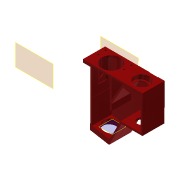
# Autodesk Inventor part: cellSTORM_v5_opticalstage
Saved by Autodesk Inventor 2022 (Build 260153000, 153)
## iProperties
Created: 2020-04-25
Part Number: cellSTORM_v5_opticalstage
Material: Generic
Document SubType Name: Modeling
Designer: diederichbenedict
Density: 1 g/cm^3
Appearance: Red
Author: diederichbenedict
Autodesk Inventor part; units mm, degrees
ref_plane "Work Plane1" through (0, 0, 0) normal (0, 0, 1) x (1, 0, 0)
ref_plane "Work Plane2" through (79.8747, 18.9526, -58.9639) normal (0, 0.0044332, 0.9999902) x (1, 0, 0)
sketch "Sketch2" plane through (79.8747, 18.9526, -58.9639) normal (0, 0.0044332, 0.9999902) x (1, 0, 0)
  line L0 (-7.3391, -43.0706) -> (-11.3391, -43.0706)
  line L1 (-7.3391, -43.0706) -> (-3.3391, -43.0706) construction
  line L2 (-11.3391, -43.0706) -> (-11.3391, -85.3324)
  line L3 (-11.3391, -85.3324) -> (19.5839, -90.7849)
  line L4 (39.6609, -51.3324) -> (73.6609, -51.3324)
  line L5 (-28.496, 8.6676) -> (-11.3391, 8.6676)
  line L6 (-11.3391, 8.6676) -> (-11.3391, -43.0706)
  line L7 (19.5839, -90.7849) -> (39.6609, -51.3324)
  line L8 (-28.496, 8.6676) -> (73.6609, 8.6676)
  line L9 (73.6609, 8.6676) -> (73.6609, -51.3324)
  line L10 (-7.2559, -79.452) -> (-8.211, -84.8684)
  line L11 (17.7582, -83.8627) -> (16.8031, -89.2791)
  line L12 (38.3797, -66.8653) -> (38.3797, -46.8653) projected
  line L13 (-11.3391, 8.6676) -> (-23.3391, 8.6676)
  line L14 (-23.3391, 8.6676) -> (-23.3391, 3.6676)
  line L15 (-23.3391, 3.6676) -> (-11.3391, 3.6676)
  line L16 (-11.3391, 3.6676) -> (-11.3391, 8.6676)
  ellipse E0 centre (54.5234, 5.3365) end of major axis (42.0164, 7.5419) minor radius 0.0004 projected
  ellipse E1 centre (3.9219, -87.5114) end of major axis (-8.339, -85.3495) minor radius 0.0004 projected
  point P0 (-79.8747, -19.2138)
  point P1 (-11.3391, 3.6676)
  point P2 (-23.3391, 8.6676)
  dimension "d0" = 4
  dimension "d1" = 180
  dimension "d156" = 3
  dimension "d157" = 3
  dimension "d158" = 1
  dimension "d159" = 94
  dimension "d160" = 85
  dimension "d161" = 60
  dimension "d163" = 34
  dimension "d180" = 12
  dimension "d181" = 5
  constraints: 32 end point, 5 horizontal, 3 parallel, 2 collinear, 2 perpendicular, 1 vertical, 9 other
  measures "d0" distance of L0.start L0.end
  measures "d1" angle of L0 L1
  measures "d156" distance from line of L2.end L10
  measures "d157" distance from line of L3.end L11
  measures "d158" distance from line of L3 L11.end
  measures "d159" distance from line of L8 L2.end
  measures "d160" distance between parallel lines of L9 L6
  measures "d161" distance between parallel lines of L8 L4
  measures "d163" distance from line of L9 L4.start
  measures "d180" distance of L15.end L14.end
  measures "d181" distance of L14.end L13.end
extrude "Extrusion1" add sketch "Sketch2" along normal blind 4 contours L6 L8 L9 L4 L7 L3 L2 | L15 L14 L5 L6 | E0 | E1
sketch "Sketch3" plane through (79.8747, 18.9703, -54.964) normal (0, 0.0044332, 0.9999902) x (1, 0, 0)
  line L0 (73.6609, 8.6676) -> (-23.3391, 8.6676) projected
  line L1 (-11.3391, 3.6676) -> (-11.3391, -85.3324) projected
  line L2 (-11.3391, -85.3324) -> (19.5839, -90.7849) projected
  line L3 (19.5839, -90.7849) -> (39.6609, -51.3324) projected
  line L4 (39.6609, -51.3324) -> (73.6609, -51.3324) projected
  line L5 (73.6609, -51.3324) -> (73.6609, 8.6676) projected
  line L6 (70.6609, 5.6676) -> (-8.3391, 5.6676)
  line L7 (-8.3391, 5.6676) -> (-8.3391, -82.8151)
  line L8 (-8.3391, -82.8151) -> (17.9175, -87.4448)
  line L9 (17.9175, -87.4448) -> (37.8215, -48.3324)
  line L10 (37.8215, -48.3324) -> (70.6609, -48.3324)
  line L11 (70.6609, -48.3324) -> (70.6609, 5.6676)
  line L12 (20.3299, 5.6676) -> (20.3299, -36.4597)
  line L13 (20.3299, -36.4597) -> (44.6523, 5.6676)
  line L14 (41.1882, 5.6676) -> (23.3299, -25.2636)
  line L15 (23.3299, -25.2636) -> (23.3299, 5.6676)
  line L16 (50.5927, -0.5756) -> (7.6402, -74.9707)
  line L17 (-23.3391, 8.6676) -> (-23.3391, 3.6676) projected
  line L18 (-23.3391, 3.6676) -> (-11.3391, 3.6676) projected
  line L19 (23.3299, -31.2636) -> (23.3299, -41.2636)
  line L20 (23.3299, -41.2636) -> (20.3299, -41.2636)
  line L21 (20.3299, -41.2636) -> (20.3299, -36.4597)
  point P0 (-79.8747, -19.2138)
  point P1 (-36.2088, 5.0266)
  dimension "d165" = 3
  dimension "d166" = 3
  dimension "d167" = 3
  dimension "d211" = 10
  constraints: 28 end point, 5 point on line, 3 perpendicular, 2 parallel, 2 vertical, 8 other
  measures "d165" distance between parallel lines of L5 L11
  measures "d166" distance between parallel lines of L12 L15
  measures "d167" distance between parallel lines of L13 L14
  measures "d211" distance of L19.start L19.end
extrude "Extrusion2" add sketch "Sketch3" along normal blind 32 contours L5 L4 L3 L2 L1 L18 L17 L0 | L13 L12 L6 L15 L14 | L19 L20 L21 L13
ref_plane "Work Plane3" through (51.6835, -64.2382, -58.0722) normal (0.309017, 0.9510565, 0) x (-0.6726294, 0.2185505, 0.7069691)
ref_plane "Work Plane4" through (49.8294, -69.9446, -58.0722) normal (-0.309017, -0.9510565, 0) x (0.6723676, -0.2184655, 0.7072444)
sketch "Sketch7" plane through (51.6691, -60.1991, -22.6127) normal (0.1736475, 0.9847982, -0.0043659) x (0.9848079, -0.1736458, 0.0007698)
  circle A0 centre (33.264, 17.4442) radius 12
  ellipse E0 centre (33.0632, 17.4064) end of major axis (45.5132, 17.4064) minor radius 12.45 projected
  point P0 (-61.32, -22.8793)
  dimension "d33" = 24
  constraints: 1 centre point
  measures "d33" diameter of A0
extrude "Extrusion5" cut sketch "Sketch7" against normal blind 5 contours A0
ref_plane "Work Plane5" through (122.0405, 25.1021, -58.0722) normal (-0.309017, -0.9510565, 0) x (0.6723676, -0.2184655, 0.7072444)
sketch "Sketch11" plane through (47.2299, 24.6379, -54.9891) normal (0, 0.9999902, -0.0044332) x (1, 0, 0)
  circle A0 centre (37.6585, -14.4614) radius 15.35
  circle A1 centre (-11.9932, -35.7166) radius 13.9 projected
  point P0 (-47.2299, -54.8793)
  dimension "d43" = 30.7
  constraints: 1 centre point
  measures "d43" diameter of A0
extrude "Extrusion9" cut sketch "Sketch11" along normal mid plane 60 contours A0
ref_plane "Arbeitsebene11" through (104.1095, -44.1462, -23.1152) normal (0, -1, 0) x (1, 0, 0)
sketch "Sketch21" plane through (104.1095, -44.1462, -23.1152) normal (0, -1, 0) x (1, 0, 0)
  ellipse E0 centre (30.7788, -17.1459) end of major axis (28.2788, -17.1459) minor radius 2.5 projected
  circle A0 centre (30.7788, -17.1459) radius 7.5
  point P0 (-104.1095, 23.1152)
  dimension "d214" = 15
  constraints: 1 centre point, 1 coincident, 1 other
  measures "d214" diameter of A0
extrude "Extrusion17" cut sketch "Sketch21" against normal blind 15 contours E0 | A0
sketch "Sketch22" plane through (68.5356, -66.3789, -58.5856) normal (-1, 0, 0) x (0, 0.0044332, 0.9999902)
  line L0 (0, 89) -> (0, 0) projected
  line L1 (0, 0) -> (36, 0) projected
  line L2 (4, 109.1334) -> (4, 78) projected
  line L3 (4, 59.5268) -> (36, 59.5268) projected
  line L4 (4, 78) -> (36, 59.5268)
  line L5 (36, 59.5268) -> (4, 59.5268)
  line L6 (4, 78) -> (4, 0) projected
  line L7 (4, 59.5268) -> (4, 78)
  line L8 (36, 89) -> (36, 0) projected
  line L9 (36, 89) -> (0, 89) projected
  point P0 (58.8793, 66.1185)
  constraints: 6 end point, 1 perpendicular
extrude "Extrusion18" add sketch "Sketch22" against normal blind 2 contours L4 L3 L6
sketch "Skizze26" plane through (79.8747, 18.9526, -58.9639) normal (0, -0.0044332, -0.9999902) x (-1, 0, 0)
  circle A0 centre (-56.1499, 7.231) radius 1.75 projected
  circle A1 centre (-56.1499, -2.769) radius 1.75 projected
  circle A2 centre (-56.1499, -12.769) radius 1.75 projected
  circle A3 centre (-56.1499, -22.769) radius 1.75 projected
  point P0 (79.8747, -19.2138)
hole "Bohrung4" at (136.0246, 26.1835, -58.996) direction (0, 0.0044332, 0.9999902) diameter 2.8 depth 12 tip angle 118
pattern_linear "Rechteckige Anordnung1" count 12 spacing 12.5 along (0, -0.9999902, 0.0044332) of "Bohrung4"
sketch "Skizze28" plane through (79.8747, 18.9526, -58.9639) normal (0, -0.0044332, -0.9999902) x (-1, 0, 0)
  line L0 (-50.0499, -35.324) -> (-50.0499, -2.924) projected
  line L1 (-62.0499, -35.324) -> (-62.0499, -2.924) projected
  line L2 (-49.0499, 19.5051) -> (-63.0499, 19.5051)
  line L3 (-63.0499, 19.5051) -> (-63.0499, -40.5846)
  line L4 (-63.0499, -40.5846) -> (-49.0499, -40.5846)
  line L5 (-49.0499, -40.5846) -> (-49.0499, 19.5051)
  point P0 (79.8747, -19.2138)
  dimension "d134" = 1
  dimension "d135" = 1
  constraints: 8 end point, 2 parallel, 1 horizontal, 1 perpendicular
  measures "d134" distance between parallel lines of L0 L5
  measures "d135" distance between parallel lines of L3 L1
extrude "Extrusion21" cut sketch "Skizze28" against normal blind 0.5
sketch "Skizze30" plane through (71.5356, -63.8439, -54.5968) normal (0.1736475, 0.9847982, -0.0043659) x (0.9848079, -0.1736458, 0.0007698)
  circle A0 centre (13.091, -14.5558) radius 12 projected
  line L0 (-2.5173, -32) -> (28.8827, -32) projected
  line L1 (27.091, 2.8884) -> (-0.909, 2.8884)
  line L2 (-0.909, 2.8884) -> (-0.909, -32)
  line L3 (-0.909, -32) -> (27.091, -32)
  line L4 (27.091, -32) -> (27.091, 2.8884)
  line L5 (27.091, 2.8884) -> (-0.909, -32) construction
  line L6 (-0.909, 2.8884) -> (27.091, -32) construction
  circle A1 centre (13.091, -14.5558) radius 12.75
  point P0 (-81.493, -54.8793)
  point P1 (27.091, -32)
  dimension "d168" = 28
  dimension "d171" = 25.5
  constraints: 12 end point, 2 midpoint, 2 parallel, 1 centre point, 1 coincident, 1 horizontal, 1 perpendicular, 1 point on line
  measures "d168" distance of L3.end L2.end
  measures "d171" diameter of A1
extrude "Extrusion23" add sketch "Skizze30" along normal blind 5 contours L2 L1 L4 L0
sketch "Skizze31" plane through (79.8747, 18.9703, -54.964) normal (0, 0.0044332, 0.9999902) x (1, 0, 0)
  line L0 (19.2086, -82.5953) -> (18.5846, -86.1339) projected
  line L1 (18.5846, -86.1339) -> (37.8215, -48.3324) projected
  line L2 (37.8215, -48.3324) -> (70.6609, -48.3324) projected
  line L3 (70.6609, -48.3324) -> (70.6609, 5.6676) projected
  line L4 (70.6609, 5.6676) -> (44.6523, 5.6676) projected
  line L5 (44.6523, 5.6676) -> (23.3299, -31.2636) projected
  line L6 (20.3299, -41.2636) -> (20.3299, 5.6676) projected
  line L7 (20.3299, 5.6676) -> (10.1606, 5.6676) projected
  line L8 (10.1606, 5.6676) -> (10.1606, -24.3324) projected
  line L9 (10.1606, -24.3324) -> (-0.1332, -24.3324) projected
  line L10 (-0.1332, -24.3324) -> (-0.1332, 5.6676) projected
  line L11 (-0.1332, 5.6676) -> (-8.3391, 5.6676) projected
  line L12 (-8.3391, 5.6676) -> (-8.3391, -77.7379) projected
  line L13 (-8.3391, -77.7379) -> (19.2086, -82.5953) projected
  circle A0 centre (56.1499, -30.269) radius 1.4 projected
  circle A1 centre (56.1499, -17.769) radius 1.4 projected
  circle A2 centre (56.1499, -5.269) radius 1.4 projected
  line L14 (-3.3391, -73.5424) -> (-3.3391, -29.3324)
  line L15 (-3.3391, -29.3324) -> (15.1606, -29.3324)
  line L16 (15.1606, -29.3324) -> (15.1606, 0.6676)
  line L17 (15.1606, 0.6676) -> (15.3299, 0.6676)
  line L18 (15.3299, 0.6676) -> (15.3299, -55.1198)
  line L19 (15.3299, -55.1198) -> (47.539, 0.6676)
  line L20 (47.539, 0.6676) -> (65.6609, 0.6676)
  line L21 (65.6609, 0.6676) -> (65.6609, -43.3324)
  line L22 (65.6609, -43.3324) -> (34.7558, -43.3324)
  line L23 (34.7558, -43.3324) -> (17.5112, -77.2189)
  line L24 (17.5112, -77.2189) -> (-3.3391, -73.5424)
  circle A3 centre (56.1499, -42.769) radius 1.4 projected
  line L25 (23.3299, -31.2636) -> (23.3299, -41.2636) projected
  line L26 (23.3299, -41.2636) -> (20.3299, -41.2636) projected
  point P0 (-79.8747, -19.2138)
  dimension "d172" = 5
  constraints: 22 end point, 10 other
  measures "d172" distance between parallel lines of L12 L14
hole "Bohrung5" at (76.5356, -10.3617, -54.8339) at (95.0352, -10.3617, -54.8339) direction (0, -0.0044332, -0.9999902) diameter 3 end through all
sketch "Skizze32" plane through (56.5356, 27.7798, -23.0027) normal (0, 0.9999902, -0.0044332) x (1, 0, 0)
  line L0 (86.3889, 36) -> (86.3889, 35.5) projected
  line L1 (86.3889, 35.5) -> (72.3889, 35.5) projected
  line L2 (72.3889, 35.5) -> (72.3889, 36) projected
  line L3 (72.3889, 36) -> (0, 36) projected
  line L4 (0, 36) -> (0, 0) projected
  line L5 (97, 0) -> (0, 0) projected
  line L6 (97, 36) -> (97, 0) projected
  line L7 (97, 36) -> (86.3889, 36) projected
  circle A0 centre (28.3527, 17.5386) radius 15.35 projected
  circle A1 centre (5.9968, 30.9932) radius 1.4
  circle A2 centre (5.9968, 18.9932) radius 1.4
  circle A3 centre (47.9968, 18.9932) radius 1.4
  circle A4 centre (47.9968, 30.9932) radius 1.4
  point P0 (-56.5356, -22.8793)
  dimension "d182" = 2.8
  dimension "d183" = 2.8
  dimension "d185" = 2.8
  dimension "d186" = 2.8
  dimension "d187" = 12
  dimension "d188" = 12
  dimension "d189" = 0
  dimension "d190" = 42
  dimension "d191" = 0
  dimension "d192" = 0
  constraints: 4 centre point
  measures "d182" diameter of A1
  measures "d183" diameter of A2
  measures "d185" diameter of A3
  measures "d186" diameter of A4
  measures "d187" distance of A4.centre A3.centre
  measures "d188" distance of A2.centre A1.centre
  measures "d189" vertical distance of A4.centre A1.centre
  measures "d190" distance of A4.centre A1.centre
  measures "d191" horizontal distance of A3.centre A4.centre
  measures "d192" horizontal distance of A2.centre A1.centre
extrude "Extrusion24" cut sketch "Skizze32" against normal blind 20 contours A1 | A2 | A3 | A4
sketch "Skizze34" plane through (79.8747, 19.1122, -22.9643) normal (0, 0.0044332, 0.9999902) x (1, 0, 0)
  line L0 (-23.3391, 8.6676) -> (-23.3391, 3.6676) projected
  line L1 (-23.3391, 3.6676) -> (-11.3391, 3.6676) projected
  line L2 (-11.3391, 3.6676) -> (-11.3391, -85.3324) projected
  line L3 (-11.3391, -85.3324) -> (19.5839, -90.7849) projected
  line L4 (19.5839, -90.7849) -> (39.6609, -51.3324) projected
  line L5 (39.6609, -51.3324) -> (73.6609, -51.3324) projected
  line L6 (73.6609, -51.3324) -> (73.6609, 8.6676) projected
  line L7 (73.6609, 8.6676) -> (-23.3391, 8.6676) projected
  line L8 (23.3299, -25.2636) -> (23.3299, 5.6676) projected
  line L9 (23.3299, 5.6676) -> (41.1882, 5.6676) projected
  line L10 (41.1882, 5.6676) -> (23.3299, -25.2636) projected
  line L11 (18.5846, -86.1339) -> (19.2086, -82.5953) projected
  line L12 (-8.3391, -77.7379) -> (19.2086, -82.5953) projected
  line L13 (-8.3391, -77.7379) -> (-8.3391, 5.6676) projected
  line L14 (-8.3391, 5.6676) -> (20.3299, 5.6676) projected
  line L15 (20.3299, 5.6676) -> (20.3299, -41.2636) projected
  line L16 (23.3299, -31.2636) -> (44.6523, 5.6676) projected
  line L17 (44.6523, 5.6676) -> (70.6609, 5.6676) projected
  line L18 (70.6609, 5.6676) -> (70.6609, -48.3324) projected
  line L19 (70.6609, -48.3324) -> (37.8215, -48.3324) projected
  line L20 (37.8215, -48.3324) -> (18.5846, -86.1339) projected
  line L21 (70.6609, 5.6676) -> (70.6609, -48.3324) projected
  line L22 (20.3299, -41.2636) -> (23.3299, -41.2636) projected
  line L23 (23.3299, -41.2636) -> (23.3299, -31.2636) projected
  ellipse E0 centre (53.5684, -0.0799) end of major axis (66.0754, -2.2852) minor radius 0.0004 projected
  line L24 (70.6609, -3.7406) -> (41.8024, 0.7315)
  point P0 (-79.8747, -19.2138)
  dimension "d213" = 1
  constraints: 2 end point, 2 point on line
  measures "d213" distance from line of E0.centre L24
extrude "Extrusion25" add sketch "Skizze34" against normal up to surface (32 mm away) contours L24 L16 L17 L18
sketch "Skizze35" plane through (122.1669, 19.7678, -22.9672) normal (-0.1531354, -0.9881955, 0.0043809) x (0.9882052, -0.1531339, 0.0006789)
  circle A0 centre (11.5094, -17.485) radius 12.7
  circle A1 centre (11.5094, -17.485) radius 10
  ellipse E0 centre (11.2506, -17.4838) end of major axis (11.2318, -29.9338) minor radius 12.4473 projected
  point P0 (-117.6833, 22.8793)
  dimension "d204" = 25.4
  dimension "d205" = 20
  constraints: 2 centre point, 1 coincident, 1 other
  measures "d204" diameter of A0
  measures "d205" diameter of A1
extrude "Extrusion26" cut sketch "Skizze35" against normal blind 1 contours A1
sketch "Skizze36" plane through (133.6936, 18.916, -40.4486) normal (-0.1531354, -0.9881955, 0.0043809) x (0.988205, -0.1531368, 0)
  circle A0 centre (0, 0) radius 10 projected
  circle A1 centre (0, 0) radius 12.7
  point P0 (-129.22, 40.2766)
  dimension "d208" = 25.4
  constraints: 1 centre point, 1 coincident
  measures "d208" diameter of A1
extrude "Extrusion27" cut sketch "Skizze36" against normal through all contours A0 | A1
sketch "Skizze37" plane through (79.8747, 19.1122, -22.9643) normal (0, 0.0044332, 0.9999902) x (1, 0, 0)
  line L0 (-23.3391, 8.6676) -> (-23.3391, 3.6676) projected
  line L1 (-23.3391, 3.6676) -> (-11.3391, 3.6676) projected
  line L2 (-11.3391, 3.6676) -> (-11.3391, -85.3324) projected
  line L3 (-11.3391, -85.3324) -> (19.5839, -90.7849) projected
  line L4 (19.5839, -90.7849) -> (39.6609, -51.3324) projected
  line L5 (39.6609, -51.3324) -> (73.6609, -51.3324) projected
  line L6 (73.6609, -51.3324) -> (73.6609, 8.6676) projected
  line L7 (73.6609, 8.6676) -> (-23.3391, 8.6676) projected
  line L8 (23.3299, -25.2636) -> (23.3299, 5.6676) projected
  line L9 (23.3299, 5.6676) -> (41.1882, 5.6676) projected
  line L10 (41.1882, 5.6676) -> (23.3299, -25.2636) projected
  line L11 (18.5846, -86.1339) -> (19.2086, -82.5953) projected
  line L12 (-8.3391, -77.7379) -> (19.2086, -82.5953) projected
  line L13 (-8.3391, -77.7379) -> (-8.3391, 5.6676) projected
  line L14 (-8.3391, 5.6676) -> (20.3299, 5.6676) projected
  line L15 (20.3299, 5.6676) -> (20.3299, -41.2636) projected
  line L16 (20.3299, -41.2636) -> (23.3299, -41.2636) projected
  line L17 (23.3299, -41.2636) -> (23.3299, -31.2636) projected
  line L18 (23.3299, -31.2636) -> (41.8024, 0.7315) projected
  line L19 (41.8024, 0.7315) -> (70.6609, -3.7406) projected
  line L20 (70.6609, -3.7406) -> (70.6609, -48.3324) projected
  line L21 (70.6609, -48.3324) -> (37.8215, -48.3324) projected
  line L22 (37.8215, -48.3324) -> (18.5846, -86.1339) projected
  line L23 (2.7914, -27.2537) -> (0.2414, -27.2537) projected
  line L24 (2.5137, -80.1552) -> (2.5137, 0.7256)
  line L25 (7.5137, -74.9442) -> (7.5137, 0.7256)
  line L26 (-8.7546, -38.7003) -> (20.7454, -38.7003)
  line L27 (20.7454, -38.7003) -> (20.7454, -31.2003)
  line L28 (20.7454, -31.2003) -> (-8.7546, -31.2003)
  line L29 (-8.7546, -31.2003) -> (-8.7546, -38.7003)
  line L30 (-8.7546, -38.7003) -> (20.7454, -31.2003) construction
  line L31 (20.7454, -38.7003) -> (-8.7546, -31.2003) construction
  point P0 (-79.8747, -19.2138)
  point P1 (5.9954, -34.9503)
  point P2 (-8.3391, -38.7003)
  point P3 (2.5137, -79.6515)
  point P4 (2.5137, -38.7003)
  dimension "d215" = 29.5
  dimension "d216" = 7.5
  constraints: 16 end point, 2 midpoint, 2 parallel, 2 vertical, 1 horizontal, 1 perpendicular, 4 other
  measures "d215" distance of L28.end L27.end
  measures "d216" distance of L27.end L26.end
extrude "Extrusion28" cut sketch "Skizze37" against normal up to surface (32 mm away) contours L12 L13 L26 L24 | L26 L13 L28 L24 | L24 L28 L25 L26 | L26 L29 L28 L13 | L25 L28 L15 L26 | L15 L28 L27 L26
body "Solid1"
